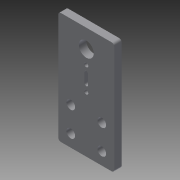
# Autodesk Inventor part: Plaque support
Saved by Autodesk Inventor 2015 SP1 (Build 190203100, 203)
## iProperties
Created: 2015-04-11
Part Number: Plaque support
Material: Generic
Document SubType Name: Modeling
Designer: Cyril
Density: 1 g/cm^3
Appearance: Default
Author: Cyril
Autodesk Inventor part; units mm, degrees
ref_plane "YZ Plane" through (0, 0, 0) normal (1, 0, 0) x (0, 1, 0)
ref_plane "XZ Plane" through (0, 0, 0) normal (0, 1, 0) x (-1, 0, 0)
ref_plane "XY Plane" through (0, 0, 0) normal (0, 0, 1) x (1, 0, 0)
sketch "Sketch1" plane through (0, 0, 0) normal (0, 0, 1) x (1, 0, 0)
  line L0 (-22.5, 45) -> (22.5, 45)
  line L1 (22.5, 45) -> (22.5, -45)
  line L2 (22.5, -45) -> (-22.5, -45)
  line L3 (-22.5, -45) -> (-22.5, 45)
  line L4 (-22.5, 45) -> (22.5, -45) construction
  line L5 (22.5, 45) -> (-22.5, -45) construction
  circle A0 centre (-12.5, -15) radius 3.5
  circle A1 centre (-12.5, -35) radius 3.5
  circle A2 centre (12.5, -35) radius 3.5
  circle A3 centre (12.5, -15) radius 3.5
  circle A4 centre (0, 30) radius 6
  line L6 (0, 45) -> (0, -45) construction
  circle A5 centre (0, 0) radius 1.65
  circle A6 centre (0, 19) radius 1.65
  line L7 (0, 0) -> (0, 19) construction
  line L8 (0, 13.3) -> (0, 5.7) construction
  line L9 (-1.5, 13.3) -> (-1.5, 5.7)
  line L10 (1.5, 5.7) -> (1.5, 13.3)
  arc A7 (1.5, 13.3) -> (-1.5, 13.3) centre (0, 13.3) ccw
  arc A8 (-1.5, 5.7) -> (1.5, 5.7) centre (0, 5.7) ccw
  point P0 (0, 0)
  point P1 (0, 9.5)
  point P2 (0, 9.5)
  dimension "d2" = 90
  dimension "d3" = 45
  dimension "d4" = 7
  dimension "d5" = 7
  dimension "d6" = 7
  dimension "d7" = 7
  dimension "d9" = 10
  dimension "d10" = 25
  dimension "d11" = 20
  dimension "d12" = 12
  dimension "d13" = 15
  dimension "d17" = 3.3
  dimension "d18" = 3.3
  dimension "d19" = 19
  dimension "d20" = 7.6
  dimension "d21" = 3
  constraints: 24 end point, 9 centre point, 8 midpoint, 4 point on circle, 4 point on line, 4 tangent, 3 parallel, 2 horizontal alignment, 2 vertical alignment, 1 coincident, 1 horizontal, 1 perpendicular, 1 symmetric about line
  measures "d2" distance of L2.end L0.start
  measures "d3" distance of L0.start L0.end
  measures "d4" diameter of A0
  measures "d5" diameter of A1
  measures "d6" diameter of A3
  measures "d7" diameter of A2
  measures "d9" distance from line of A1.centre L2
  measures "d10" distance of A2.centre A1.centre
  measures "d11" distance of A1.centre A0.centre
  measures "d12" diameter of A4
  measures "d13" distance from line of L0 A4.centre
  measures "d17" diameter of A5
  measures "d18" diameter of A6
  measures "d19" distance of L7.start L7.end
  measures "d20" distance of L10.start L10.end
  measures "d21" distance between parallel lines of L9 L10
extrude "Extrusion3" add sketch "Sketch1" along normal blind 6
fillet "Fillet2" radius 2 4 edges at (-22.5, 45, 3) (-22.5, -45, 3) (22.5, -45, 3) (22.5, 45, 3)
equation "\"d5\" = d4"
equation "\"d6\" = d4"
equation "\"d7\" = d4"
equation "\"d18\" = d17"
body "Solid3"
